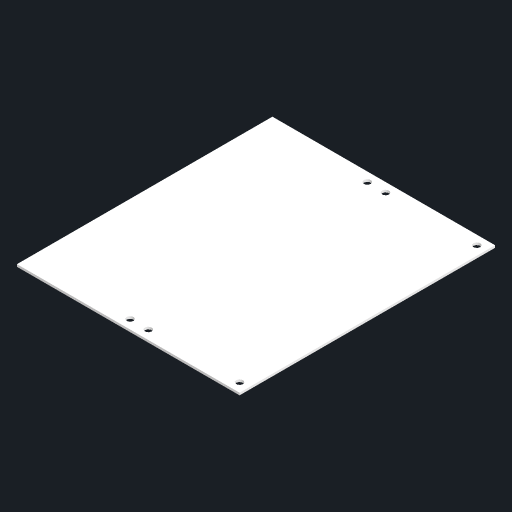
# Autodesk Inventor part: intake
Saved by Autodesk Inventor 2023 (Build 270158000, 158)
## iProperties
Created: 2023-04-09
Part Number: intake
Material: ABS Plastic
Document SubType Name: Modeling
Designer: Windows Macbook
Density: 1.06 g/cm^3
Appearance: Smooth - White
Author: Windows Macbook
Autodesk Inventor part; units mm, degrees
ref_plane "YZ Plane" through (0, 0, 0) normal (1, 0, 0) x (0, 1, 0)
ref_plane "XZ Plane" through (0, 0, 0) normal (0, 1, 0) x (-1, 0, 0)
ref_plane "XY Plane" through (0, 0, 0) normal (0, 0, 1) x (1, 0, 0)
sketch "Sketch1" plane through (0, 0, 0) normal (0, 1, 0) x (-1, 0, 0)
  line L0 (0, 0) -> (0, -177.8)
  line L1 (0, 0) -> (154.94, 0)
  line L2 (154.94, 0) -> (154.94, -177.8)
  line L3 (154.94, -177.8) -> (0, -177.8)
  dimension "d0" = 177.8
  dimension "d1" = 154.94
  dimension "d2" = 177.8
  constraints: 8 end point, 1 horizontal, 1 perpendicular, 1 vertical
  measures "d0" distance of L0.start L0.end
  measures "d1" distance of L0.start L1.end
  measures "d2" distance of L1.end L2.end
extrude "Extrusion1" add sketch "Sketch1" along normal blind 1.5875
sketch "Sketch2" plane through (0, 1.5875, 0) normal (0, 1, 0) x (1, 0, 0)
  line L0 (-154.94, 0) -> (0, 0) projected
  line L1 (-154.94, 0) -> (-145.9597, 0) construction
  line L2 (0, 177.8) -> (-154.94, 177.8) projected
  line L3 (-154.94, 177.8) -> (-145.9597, 177.8) construction
  line L4 (0, 0) -> (0, 177.8) projected
  line L5 (0, 177.8) -> (-12.7, 177.8)
  line L6 (-12.7, 177.8) -> (0, 165.1)
  line L7 (0, 177.8) -> (-6.35, 171.45)
  line L8 (0, 177.8) -> (8.9803, 177.8) construction
  line L9 (0, 0) -> (-12.7, 0)
  line L10 (-12.7, 0) -> (0, 12.7)
  line L11 (0, 0) -> (-6.35, 6.35)
  line L12 (-6.35, 171.45) -> (-69.85, 171.45)
  line L13 (-69.85, 171.45) -> (-82.55, 171.45)
  line L14 (-6.35, 6.35) -> (-69.85, 6.35)
  line L15 (-6.35, 6.35) -> (57.15, 6.35) construction
  line L16 (-69.85, 6.35) -> (-82.55, 6.35)
  dimension "d18" = 12.7
  dimension "d19" = 45
  dimension "d20" = 135
  dimension "d21" = 12.7
  dimension "d22" = 63.5
  dimension "d23" = 12.7
  dimension "d24" = 63.5
  dimension "d25" = 180
  dimension "d26" = 12.7
  constraints: 28 end point, 6 coincident, 6 horizontal, 5 point on line, 2 equal length, 2 midpoint
  measures "d18" distance of L2.start L5.end
  measures "d19" angle of L6 L5
  measures "d20" angle of L7 L8
  measures "d21" distance of L0.end L9.end
  measures "d22" distance of L12.start L12.end
  measures "d23" distance of L12.end L13.end
  measures "d24" distance of L11.end L14.end
  measures "d25" angle of L14 L15
  measures "d26" distance of L14.end L16.end
hole "Hole2" at (-6.35, 1.5875, -6.35) at (-6.35, 1.5875, -171.45) at (-69.85, 1.5875, -171.45) at (-82.55, 1.5875, -171.45) at (-69.85, 1.5875, -6.35) at (-82.55, 1.5875, -6.35) direction (0, -1, 0) diameter 4.7625 end through all
body "Solid1"
